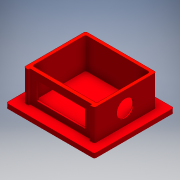
# Autodesk Inventor part: integratedSampleHolder_xyBase
Saved by Autodesk Inventor 2016 (Build 200138000, 138)
## iProperties
Created: 2016-10-05
Part Number: integratedSampleHolder_xyBase
Material: Generic
Document SubType Name: Modeling
Designer: sims01
Density: 1 g/cm^3
Appearance: Default
Author: sims01
Autodesk Inventor part; units mm, degrees
ref_plane "YZ Plane" through (0, 0, 0) normal (1, 0, 0) x (0, 1, 0)
ref_plane "XZ Plane" through (0, 0, 0) normal (0, 1, 0) x (-1, 0, 0)
ref_plane "XY Plane" through (0, 0, 0) normal (0, 0, 1) x (1, 0, 0)
sketch "Sketch1" plane through (0, 0, 0) normal (0, 0, 1) x (1, 0, 0)
  line L0 (-38, 35) -> (38, 35)
  line L1 (40, 33) -> (40, -33)
  line L2 (38, -35) -> (-38, -35)
  line L3 (-40, -33) -> (-40, 33)
  arc A0 (-38, 35) -> (-40, 33) centre (-38, 33) ccw
  arc A1 (-40, -33) -> (-38, -35) centre (-38, -33) ccw
  arc A2 (38, -35) -> (40, -33) centre (38, -33) ccw
  arc A3 (40, 33) -> (38, 35) centre (38, 33) ccw
  point P0 (0, 0)
  point P1 (-40, 35)
  point P2 (40, 35)
  point P3 (-40, -35)
  dimension "d0" = 80
  dimension "d1" = 70
  dimension "d2" = 35
  dimension "d3" = 40
  dimension "d4" = 2
  constraints: 8 end point, 8 point on circle, 8 tangent, 6 point on line, 4 centre point, 3 equal radius, 2 parallel, 1 horizontal, 1 perpendicular
  measures "d0" distance of point (-40, 35) point (40, 35)
  measures "d1" distance of point (-40, -35) point (-40, 35)
  measures "d2" distance from line of L0 point (0, 0)
  measures "d3" distance from line of point (0, 0) L1
  measures "d4" radius of A0
extrude "base" add sketch "Sketch1" along normal blind 5
sketch "Sketch2" plane through (0, 0, 5) normal (0, 0, 1) x (1, 0, 0)
  line L0 (-38, 35) -> (38, 35)
  line L1 (40, 33) -> (40, -33)
  line L2 (38, -35) -> (-38, -35)
  line L3 (-40, -33) -> (-40, 33)
  line L4 (40, -33) -> (40, 33) projected
  line L5 (38, 35) -> (-38, 35) projected
  line L6 (-40, 33) -> (-40, -33) projected
  line L7 (-38, -35) -> (38, -35) projected
  arc A0 (-38, 35) -> (-40, 33) centre (-38, 33) ccw
  arc A1 (-40, -33) -> (-38, -35) centre (-38, -33) ccw
  arc A2 (38, -35) -> (40, -33) centre (38, -33) ccw
  arc A3 (40, 33) -> (38, 35) centre (38, 33) ccw
  line L8 (-34.5, 31.5) -> (34.5, 31.5)
  line L9 (36.5, 29.5) -> (36.5, -27)
  line L10 (34.5, -29) -> (-34.5, -29)
  line L11 (-36.5, -27) -> (-36.5, 29.5)
  arc A4 (-34.5, 31.5) -> (-36.5, 29.5) centre (-34.5, 29.5) ccw
  arc A5 (-36.5, -27) -> (-34.5, -29) centre (-34.5, -27) ccw
  arc A6 (34.5, -29) -> (36.5, -27) centre (34.5, -27) ccw
  arc A7 (36.5, 29.5) -> (34.5, 31.5) centre (34.5, 29.5) ccw
  point P0 (0, 0)
  dimension "d7" = 2
  dimension "d8" = 3.5
  dimension "d9" = 3.5
  dimension "d10" = 3.5
  dimension "d12" = 2
  dimension "d123" = 6
  constraints: 16 end point, 16 point on circle, 16 tangent, 8 centre point, 6 equal radius, 4 collinear, 4 parallel, 2 horizontal, 2 perpendicular
  measures "d7" radius of A0
  measures "d8" distance between parallel lines of L3 L11
  measures "d9" distance between parallel lines of L0 L8
  measures "d10" distance between parallel lines of L1 L9
  measures "d12" radius of A4
  measures "d123" distance between parallel lines of L10 L2
extrude "walls" add sketch "Sketch2" along normal blind 35
sketch "Sketch7" plane through (0, 0, 5) normal (0, 0, 1) x (1, 0, 0)
  line L0 (34.5, -29) -> (-34.5, -29) projected
  circle A0 centre (0, -14) radius 2.875
  circle A1 centre (0, 1) radius 2.875
  circle A2 centre (-15, 1) radius 2.875
  circle A3 centre (0, 16) radius 2.875
  circle A4 centre (15, 1) radius 2.875
  point P0 (0, 0)
  dimension "d40" = 15
  dimension "d41" = 15
  dimension "d42" = 15
  dimension "d51" = 15
  dimension "d52" = 15
  dimension "d53" = 5.75
  dimension "d54" = 5.75
  dimension "d55" = 5.75
  dimension "d56" = 5.75
  dimension "d57" = 5.75
  constraints: 5 centre point, 5 coincident, 3 horizontal alignment, 3 vertical alignment
  measures "d40" distance of point (0, 1) point (0, -14)
  measures "d41" distance of point (0, 1) point (-15, 1)
  measures "d42" horizontal distance of point (15, 1) point (0, 0)
  measures "d51" distance of point (0, 16) point (0, 1)
  measures "d52" distance from line of L0 point (0, -14)
  measures "d53" diameter of A0
  measures "d54" diameter of A2
  measures "d55" diameter of A1
  measures "d56" diameter of A3
  measures "d57" diameter of A4
extrude "magnets" cut sketch "Sketch7" against normal blind 2.5
sketch "Sketch10" plane through (0, 0, 0) normal (0, 0, -1) x (-1, 0, 0)
  line L0 (-48, -45) -> (48, -45)
  line L1 (50, -43) -> (50, 43)
  line L2 (48, 45) -> (-48, 45)
  line L3 (-50, 43) -> (-50, -43)
  line L4 (38, -35) -> (-38, -35) projected
  line L5 (-40, -33) -> (-40, 33) projected
  line L6 (-38, 35) -> (38, 35) projected
  line L7 (40, 33) -> (40, -33) projected
  arc A0 (-50, -43) -> (-48, -45) centre (-48, -43) ccw
  arc A1 (48, -45) -> (50, -43) centre (48, -43) ccw
  arc A2 (50, 43) -> (48, 45) centre (48, 43) ccw
  arc A3 (-48, 45) -> (-50, 43) centre (-48, 43) ccw
  point P0 (0, 0)
  dimension "d73" = 10
  dimension "d74" = 10
  dimension "d75" = 10
  dimension "d76" = 10
  dimension "d77" = 2
  constraints: 8 end point, 8 point on circle, 8 tangent, 4 centre point, 3 equal radius, 2 parallel, 1 horizontal, 1 perpendicular
  measures "d73" distance between parallel lines of L0 L4
  measures "d74" distance between parallel lines of L5 L3
  measures "d75" distance between parallel lines of L2 L6
  measures "d76" distance between parallel lines of L1 L7
  measures "d77" radius of A0
extrude "xyStageMount" add sketch "Sketch10" against normal blind 5
sketch "Sketch15" plane through (-34.5, -29, 5) normal (0, 1, 0) x (1, 0, 0)
  line L0 (62, -27) -> (7, -27)
  line L1 (7, -27) -> (7, -7)
  line L2 (7, -7) -> (62, -7)
  line L3 (62, -7) -> (62, -27)
  line L4 (0, 0) -> (69, 0) projected
  line L5 (67, -2) -> (2, -2)
  line L6 (2, -2) -> (2, -32)
  line L7 (2, -32) -> (67, -32)
  line L8 (67, -32) -> (67, -2)
  line L9 (-13.5, 5) -> (82.5, 5) projected
  point P0 (34.5, 5)
  dimension "d107" = 20
  dimension "d108" = 55
  dimension "d109" = 27.5
  dimension "d111" = 5
  dimension "d112" = 5
  dimension "d113" = 5
  dimension "d114" = 5
  dimension "d136" = 27
  constraints: 16 end point, 4 parallel, 2 horizontal, 2 perpendicular
  measures "d107" distance of L2.end L0.start
  measures "d108" distance of L0.start L0.end
  measures "d109" distance from line of point (34.5, 5) L3
  measures "d111" distance between parallel lines of L7 L0
  measures "d112" distance between parallel lines of L5 L2
  measures "d113" distance between parallel lines of L3 L8
  measures "d114" distance between parallel lines of L6 L1
  measures "d136" distance between parallel lines of L0 L4
extrude "coverSlipWindowExt" cut sketch "Sketch15" against normal blind 2
sketch "Sketch16" plane through (-27.5, -29, 12) normal (0, 1, 0) x (1, 0, 0)
  line L0 (55, 0) -> (0, 0)
  line L1 (0, 0) -> (0, -20)
  line L2 (0, -20) -> (55, -20)
  line L3 (55, -20) -> (55, 0)
  line L4 (55, -20) -> (55, 0) projected
  line L5 (0, -20) -> (55, -20) projected
  line L6 (0, 0) -> (0, -20) projected
  line L7 (55, 0) -> (0, 0) projected
  point P0 (27.5, 12)
  constraints: 8 end point, 4 collinear, 2 parallel, 1 horizontal, 1 perpendicular
extrude "rectWindowExt" cut sketch "Sketch16" against normal up to surface (6 mm away)
sketch "Sketch17" plane through (-38, -35, 40) normal (0, -1, 0) x (1, 0, 0)
  line L0 (3, 0) -> (73, 0)
  line L1 (73, 0) -> (73, -35)
  line L2 (73, -35) -> (3, -35)
  line L3 (3, -35) -> (3, 0)
  line L4 (10.5, -8) -> (65.5, -8) projected
  line L5 (10.5, -8) -> (65.5, -8)
  line L6 (65.5, -8) -> (65.5, -28)
  line L7 (65.5, -28) -> (10.5, -28)
  line L8 (10.5, -28) -> (10.5, -8)
  line L9 (10.5, -28) -> (10.5, -8) projected
  line L10 (65.5, -28) -> (10.5, -28) projected
  line L11 (65.5, -8) -> (65.5, -28) projected
  line L12 (0, 0) -> (76, 0) projected
  line L13 (-10, -35) -> (86, -35) projected
  point P0 (38, -40)
  dimension "d120" = 70
  dimension "d121" = 35
  constraints: 16 end point, 6 collinear, 4 parallel, 2 horizontal, 2 perpendicular
  measures "d120" distance of L0.start L0.end
  measures "d121" distance from line of point (38, -40) L1
extrude "objWindowExt" cut sketch "Sketch17" against normal blind 2
sketch "Sketch18" plane through (36.5, -27, 5) normal (-1, 0, 0) x (0, 0, 1)
  circle A0 centre (17, 27) radius 15
  line L0 (0, 0) -> (0, 56.5) projected
  point P0 (-5, 27)
  dimension "d128" = 30
  dimension "d129" = 17
  constraints: 1 centre point, 1 horizontal alignment
  measures "d128" diameter of A0
  measures "d129" distance from line of L0 A0.centre
extrude "coverSlipWindowCirc" cut sketch "Sketch18" against normal blind 2
sketch "Sketch19" plane through (38.5, 0, 22) normal (-1, 0, 0) x (0, 0, 1)
  circle A0 centre (0, 0) radius 9.75
  line L0 (-17, -27) -> (-17, 29.5) projected
  circle A1 centre (0, 0) radius 15 projected
  point P0 (-22, 0)
  dimension "d133" = 19.5
  constraints: 1 centre point, 1 concentric
  measures "d133" diameter of A0
extrude "coverSlipCircExt" cut sketch "Sketch19" against normal up to next contours A0
equation "\"d2\" = 0.5 * d1"
equation "\"d3\" = 0.5 * d0"
equation "\"d9\" = d8"
equation "\"d10\" = d8"
equation "\"d41\" = d40"
equation "\"d42\" = d40"
equation "\"d51\" = d40"
equation "\"d54\" = d53"
equation "\"d55\" = d53"
equation "\"d56\" = d53"
equation "\"d57\" = d53"
equation "\"d74\" = d73"
equation "\"d75\" = d73"
equation "\"d76\" = d73"
equation "\"d109\" = 0.5 * d108"
equation "\"d112\" = d111"
equation "\"d113\" = d111"
equation "\"d114\" = d111"
equation "\"d121\" = 0.5 * d120"
body "Solid1"
